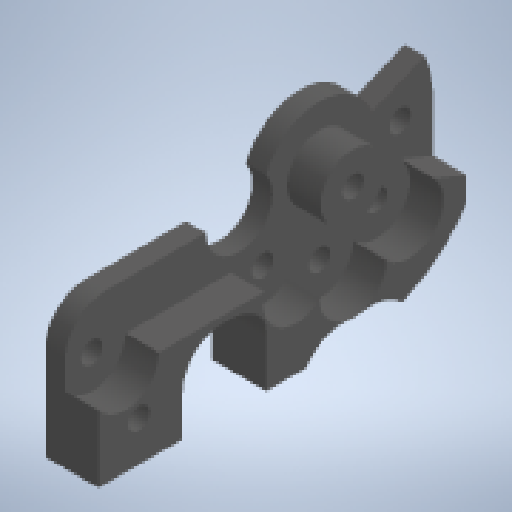
# Autodesk Inventor part: toe_springjoint_bace_under_left
Saved by Autodesk Inventor 2024.1 (Build 281209000, 209)
## iProperties
Created: 2024-02-25
Part Number: toe_springjoint_bace_under_left
Material: 一般
Document SubType Name: Modeling
Designer: hibik
Density: 1 g/cm^3
Appearance: 既定
Author: hibik
Autodesk Inventor part; units mm, degrees
ref_plane "YZ Plane" through (0, 0, 0) normal (1, 0, 0) x (0, 1, 0)
ref_plane "XZ Plane" through (0, 0, 0) normal (0, 1, 0) x (-1, 0, 0)
ref_plane "XY Plane" through (0, 0, 0) normal (0, 0, 1) x (1, 0, 0)
sketch "スケッチ1" plane through (0, 0, 0) normal (1, 0, 0) x (0, 1, 0)
  circle A0 centre (0, 0) radius 4.25
  circle A1 centre (0, 0) radius 6 construction
  circle A2 centre (6, 0) radius 0.8
  line L0 (-14, 0) -> (14, 0) projected
  circle A3 centre (4.2426, 4.2426) radius 0.8
  circle A4 centre (0, 6) radius 0.8
  circle A5 centre (-4.2426, 4.2426) radius 0.8
  circle A6 centre (-6, 0) radius 0.8
  circle A7 centre (-4.2426, -4.2426) radius 0.8
  circle A8 centre (0, -6) radius 0.8
  circle A9 centre (4.2426, -4.2426) radius 0.8
  circle A10 centre (0, 0) radius 2.4
  line L1 (0, 0) -> (0, 6)
  line L2 (0, 0) -> (2.2961, -5.5433)
  circle A11 centre (0, 0) radius 10
  line L3 (2.2961, -5.5433) -> (3.8268, -9.2388)
  line L4 (0, -9.2388) -> (-10, -9.2388)
  line L5 (-10, -9.2388) -> (-10, 20)
  line L6 (-10, 20) -> (0, 20)
  line L7 (0, 20) -> (0, -9.2388)
  line L8 (0, -6) -> (4.2426, -4.2426) construction
  line L9 (0, -9.2388) -> (3.8268, -9.2388)
  circle A12 centre (0, 6) radius 2.5
  point P0 (0, 5.2)
  point P1 (0, 6.8)
  point P2 (-10, 0)
  point P3 (2.1213, -5.1213)
  point P4 (0, 2.4)
  point P5 (0.9184, -2.2173)
  point P6 (1.4789, 3.9844)
  point P7 (0, 8.5)
  point P8 (1.6264, -3.9265)
  dimension "d0" = 8.5
  dimension "d1" = 12
  dimension "d2" = 1.6
  dimension "d5" = 360
  dimension "d7" = 4.8
  dimension "d8" = 4
  dimension "d21" = 5
  dimension "d23" = 20
  constraints: 18 end point, 12 centre point, 6 coincident, 6 point on line, 3 point on circle, 2 horizontal, 2 parallel, 1 midpoint, 1 perpendicular, 1 vertical, 20 other
  measures "d0" diameter of A0
  measures "d1" diameter of A1
  measures "d2" diameter of A2
  measures "d7" diameter of A10
  measures "d21" diameter of A12
  measures "d23" distance from line of L6 point (0, 0)
extrude "押し出し1" add sketch "スケッチ1" along normal blind 1.5 contours L0 A10 L1 A12 A0 | A0 L2 A10 L0 | L2 L3 L9 L7 A8 A0 | A0 L7 A10 L2 | A10 L2 L0 | L0 L1 A10 | L1 A10 L0 A0 A12 | L7 A8 L4 A11 L0 A6 A0 | A0 L0 A10 L7 | A10 L7 L2 | L7 A10 L0 | L0 A10 L1 | A0 L0 A6 A11 L7 A12 | A11 L4 L9 | A11 L5 L6 L7
sketch "スケッチ3" plane through (1.5, 0, 0) normal (1, 0, 0) x (0, 0, -1)
  circle A0 centre (0, 0) radius 2.5 construction
  line L0 (0, -2.5) -> (-20, -2.5) construction
  line L1 (-20, -2.5) -> (0, -2.5)
  line L2 (0, -2.5) -> (0, -3.5)
  line L3 (0, -3.5) -> (-20, -3.5)
  line L4 (-20, -3.5) -> (-20, -2.5)
  circle A1 centre (0, 0) radius 3.5
  line L5 (-20, 0) -> (-20, -10) projected
  line L6 (-8.5, 0) -> (-20, 0) projected
  line L7 (-20, 0) -> (-20, -10) projected
  line L8 (-20, -10) -> (0, -10) projected
  arc A2 (0, -10) -> (9.2388, 3.8268) centre (0, 0) ccw projected
  line L9 (9.2388, 3.8268) -> (3.9265, 1.6264) projected
  circle A3 centre (4.2426, -4.2426) radius 0.8 projected
  circle A4 centre (-4.2426, -4.2426) radius 0.8 projected
  circle A5 centre (0, -6) radius 0.8 projected
  circle A6 centre (-4.2426, -4.2426) radius 2.5
  circle A7 centre (0, -6) radius 2.5
  circle A8 centre (4.2426, -4.2426) radius 2.5
  circle A9 centre (6, 0) radius 0.8 projected
  circle A10 centre (6, 0) radius 2.5
  arc A11 (-8.5, 0) -> (-3.9844, 1.4789) centre (-6, 0) ccw projected
  arc A12 (3.9265, 1.6264) -> (-3.9844, 1.4789) centre (0, 0) ccw projected
  circle A13 centre (0, 0) radius 2.4
  line L10 (3.2336, -1.3394) -> (9.2388, -3.8268)
  line L11 (6, 0) -> (4.2426, -4.2426) construction
  point P0 (6.0349, 2.4998)
  point P1 (6.0349, -2.4998)
  point P2 (2.4998, -6.0349)
  point P3 (-2.4998, -6.0349)
  point P4 (-6.6298, -3.5)
  point P5 (5.1213, -2.1213)
  point P6 (6.0349, -2.4998)
  dimension "d13" = 5
  dimension "d14" = 1
  dimension "d15" = 5
  dimension "d16" = 5
  dimension "d17" = 5
  dimension "d18" = 5
  dimension "d22" = 4.8
  constraints: 14 end point, 8 coincident, 5 centre point, 4 horizontal, 3 point on line, 2 parallel, 1 collinear, 1 midpoint, 1 perpendicular, 1 point on circle, 1 vertical alignment, 5 other
  measures "d14" distance between parallel lines of L0 L3
  measures "d15" diameter of A6
  measures "d16" diameter of A7
  measures "d17" diameter of A8
  measures "d18" diameter of A10
  measures "d22" diameter of A13
extrude "押し出し2" add sketch "スケッチ3" along normal blind 2.5 contours L3 A6 A7 A8 L10 A2 L8 L5 | A13
sketch "スケッチ4" plane through (0, 0, 0) normal (-1, 0, 0) x (0, 0, 1)
  line L0 (3.7223, -10.4472) -> (3.446, -9.9687) projected
  arc A0 (3.446, -9.9687) -> (0.6267, -8.4769) centre (0.848, -11.4687) ccw projected
  arc A1 (-1.1087, -8.4274) -> (0.6267, -8.4769) centre (0, 0) ccw projected
  arc A2 (-1.1087, -8.4274) -> (-4.5, -11.4018) centre (-1.5, -11.4018) ccw projected
  line L1 (-4.5, -11.4018) -> (-4.5, -11.9059) projected
  arc A3 (-4.5, -11.9059) -> (-1.875, -14.8824) centre (-1.5, -11.9059) ccw projected
  arc A4 (-1.875, -14.8824) -> (1.4053, -14.934) centre (0, 0) ccw projected
  arc A5 (1.4053, -14.934) -> (3.7223, -10.4472) centre (1.1242, -11.9472) ccw projected
  arc A6 (-8.5, -16) -> (-5.5, -19) centre (-5.5, -16) ccw projected
  line L2 (-8.5, -16) -> (-8.5, 0) projected
  arc A7 (8.2057, 2.2174) -> (-8.5, 0) centre (0, 0) ccw projected
  arc A8 (8.2057, 2.2174) -> (11.1018, 0) centre (11.1018, 3) ccw projected
  line L3 (11.1018, 0) -> (16, 0) projected
  arc A9 (19, -3) -> (16, 0) centre (16, -3) ccw projected
  line L4 (19, -3) -> (19, -16) projected
  arc A10 (16, -19) -> (19, -16) centre (16, -16) ccw projected
  line L5 (16, -19) -> (-5.5, -19) projected
  circle A11 centre (-6, 0) radius 1 projected
  circle A12 centre (-4.2426, 4.2426) radius 1 projected
  circle A13 centre (0, 6) radius 1 projected
  circle A14 centre (4.2426, 4.2426) radius 1 projected
  circle A15 centre (13.8033, -13.8033) radius 0.8 projected
  circle A16 centre (-2.5, -17) radius 0.8 projected
  circle A17 centre (17, -17) radius 0.8 projected
  circle A18 centre (6, 0) radius 1 projected
  circle A19 centre (4.2426, -4.2426) radius 1 projected
  circle A20 centre (-4.2426, -4.2426) radius 1 projected
  circle A21 centre (0, -6) radius 1 projected
  circle A22 centre (0, 0) radius 4.25 projected
  circle A23 centre (17, -3.5) radius 0.8 projected
  arc A24 (12.1835, -8.75) -> (9.7468, -4) centre (9.7468, -7) ccw projected
  line L6 (9.7468, -4) -> (9.1241, -4) projected
  arc A25 (9.1241, -4) -> (6.7439, -5.1739) centre (9.1241, -7) ccw projected
  arc A26 (6.7439, -5.1739) -> (6.878, -7.913) centre (9.4761, -6.413) ccw projected
  line L7 (6.878, -7.913) -> (7.1869, -8.448) projected
  arc A27 (7.1869, -8.448) -> (12.1835, -8.75) centre (9.785, -6.948) ccw projected
  circle A28 centre (-6, 0) radius 0.8 projected
  circle A29 centre (-4.2426, -4.2426) radius 0.8 projected
  circle A30 centre (4.2426, -4.2426) radius 0.8 projected
  circle A31 centre (0, -6) radius 0.8 projected
  arc A32 (3.9844, 1.4789) -> (8.5, 0) centre (6, 0) ccw projected
  arc A33 (3.9844, 1.4789) -> (-3.9265, 1.6264) centre (0, 0) ccw projected
  line L8 (-9.2388, 3.8268) -> (-3.9265, 1.6264) projected
  arc A34 (-9.2388, 3.8268) -> (0, -10) centre (0, 0) ccw projected
  line L9 (20, -10) -> (0, -10) projected
  line L10 (20, 0) -> (20, -10) projected
  line L11 (8.5, 0) -> (20, 0) projected
  line L12 (12.7468, -10) -> (12.7468, -6.471)
  line L13 (6.4797, -10) -> (6.4797, -6.5597)
  point P0 (-3.6504, -9.3099)
  point P1 (3.4641, -10)
  point P2 (19, -10)
  point P3 (-8.5, -5.2678)
  point P4 (-7.853, 3.2528)
  point P5 (12.7468, -7)
  constraints: 4 end point, 2 point on circle, 2 point on line, 2 vertical, 1 tangent
extrude "押し出し3" cut sketch "スケッチ4" against normal through all contours L9 A34 A2 A1 A0 L0 | L13 A26 L7 A27 A24 L12 L9 | A26 A25 L6 A24 A27 L7 | L4 A9 L11 L10 L9 | A34 L8 A7 L2 | A23
sketch "スケッチ5" plane through (4, 0, 0) normal (1, 0, 0) x (0, 0, -1)
  circle A0 centre (-17, -3.5) radius 2.5
  arc A1 (-16.2, -3.5) -> (-17.8, -3.5) centre (-17, -3.5) ccw projected
  point P0 (0, 0)
  dimension "d26" = 5
  constraints: 1 centre point, 1 concentric
  measures "d26" diameter of A0
extrude "押し出し4" cut sketch "スケッチ5" against normal up to surface (2.5 mm away)
sketch "スケッチ6" plane through (4, 0, 0) normal (1, 0, 0) x (0, 0, -1)
  circle A0 centre (-16, -7) radius 0.8 projected
  circle A1 centre (0, 0) radius 0.8 projected
  point P0 (0, 0)
extrude "押し出し5" cut sketch "スケッチ6" against normal through all
